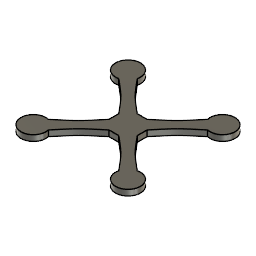
Drone 2 Polegadas (Autodesk Fusion 360 design; units mm, degrees)
Autodesk Fusion 360 part; units mm, degrees
note: some values were not read from the file. Set by a fixed rule: which sketch regions a step uses.
sketch "Esboço2" plane through (0, 0, 0) normal (0, 0, 1) x (1, 0, 0)
  circle A0 centre (-40.4, 40.4) radius 10.65
  circle A1 centre (40.4, 40.4) radius 10.65
  circle A2 centre (-40.4, -40.4) radius 10.65
  circle A3 centre (40.4, -40.4) radius 10.65
  line L0 (-40.4, 40.4) -> (-12.0945, 12.0945) construction
  line L1 (40.4, 40.4) -> (12.0945, 12.0945) construction
  line L2 (-40.4, -40.4) -> (-12.0945, -12.0945) construction
  line L3 (40.4, -40.4) -> (12.0945, -12.0945) construction
  line L4 (-6.0945, 12.0945) -> (6.0945, 12.0945)
  line L5 (12.0945, 6.0945) -> (12.0945, -6.0945)
  line L6 (6.0945, -12.0945) -> (-6.0945, -12.0945)
  line L7 (-12.0945, -6.0945) -> (-12.0945, 6.0945)
  line L8 (-30.0303, 37.9728) -> (-37.9728, 30.0303)
  line L9 (-37.9728, 30.0303) -> (-12.0945, 4.152) construction
  line L10 (-12.0945, 4.152) -> (-4.152, 12.0945) construction
  line L11 (-4.152, 12.0945) -> (-30.0303, 37.9728) construction
  line L12 (-17.0911, 25.0336) -> (-21.0624, 21.0624) construction
  spline S0 degree 2 poles (-30.0303, 37.9728) (-18.2817, 23.8431) (-4.152, 12.0945) knots 0 0 0 3.668443 3.668443 3.668443 weights 1 3 1
  spline S1 degree 2 poles (-37.9728, 30.0303) (-23.8431, 18.2817) (-12.0945, 4.152) knots 0 0 0 3.668443 3.668443 3.668443 weights 1 3 1
  line L13 (0, 12.0945) -> (0, -12.0945) construction
  spline S2 degree 2 poles (30.0303, 37.9728) (18.2817, 23.8431) (4.152, 12.0945) knots 0 0 0 3.668443 3.668443 3.668443 weights 1 3 1
  spline S3 degree 2 poles (37.9728, 30.0303) (23.8431, 18.2817) (12.0945, 4.152) knots 0 0 0 3.668443 3.668443 3.668443 weights 1 3 1
  line L14 (-12.0945, 0) -> (12.0945, 0) construction
  spline S4 degree 2 poles (-30.0303, -37.9728) (-18.2817, -23.8431) (-4.152, -12.0945) knots 0 0 0 3.668443 3.668443 3.668443 weights 1 3 1
  spline S5 degree 2 poles (-37.9728, -30.0303) (-23.8431, -18.2817) (-12.0945, -4.152) knots 0 0 0 3.668443 3.668443 3.668443 weights 1 3 1
  spline S6 degree 2 poles (30.0303, -37.9728) (18.2817, -23.8431) (4.152, -12.0945) knots 0 0 0 3.668443 3.668443 3.668443 weights 1 3 1
  spline S7 degree 2 poles (37.9728, -30.0303) (23.8431, -18.2817) (12.0945, -4.152) knots 0 0 0 3.668443 3.668443 3.668443 weights 1 3 1
  arc A4 (-6.0945, 12.0945) -> (-12.0945, 6.0945) centre (-6.0945, 6.0945) ccw
  arc A5 (12.0945, 6.0945) -> (6.0945, 12.0945) centre (6.0945, 6.0945) ccw
  arc A6 (-12.0945, -6.0945) -> (-6.0945, -12.0945) centre (-6.0945, -6.0945) ccw
  arc A7 (6.0945, -12.0945) -> (12.0945, -6.0945) centre (6.0945, -6.0945) ccw
  dimension "d49" = 80.8
  dimension "d50" = 80.8
  dimension "d51" = 21.3
  dimension "d52" = 21.3
  dimension "d53" = 21.3
  dimension "d54" = 21.3
  dimension "d55" = 114.2685
  dimension "d56" = 40.03
  dimension "d57" = 40.03
  dimension "d58" = 40.03
  dimension "d59" = 40.03
  dimension "d69" = 6
  dimension "d70" = 6
  dimension "d71" = 6
  dimension "d72" = 6
  constraint coincident A0.centre L0.start
  constraint coincident A1.centre L1.start
  constraint coincident A2.centre L2.start
  constraint coincident A3.centre L3.start
  constraint coincident A0 L8.start
  constraint coincident A0 L8.end
  constraint coincident L7 L9.end
  constraint coincident L4 L10.end
  constraint perpendicular L9 L10
  constraint coincident L0 L12.end
  constraint symmetric L0 L8.start L8.end
  constraint symmetric L0 L10.end L9.end
  constraint symmetric L0 S0 S1
  constraint perpendicular L6 L13
  constraint symmetric L8.start L13 S2.start
  constraint symmetric L10.end L13 S2.end
  constraint symmetric S0 L13 S2
  constraint symmetric L8.end L13 S3.start
  constraint symmetric L9.end L13 S3.end
  constraint symmetric S1 L13 S3
  constraint perpendicular L5 L14
  constraint symmetric L8.start L14 S4.start
  constraint symmetric L10.end L14 S4.end
  constraint symmetric S0 L14 S4
  constraint symmetric L8.end L14 S5.start
  constraint symmetric L9.end L14 S5.end
  constraint symmetric S1 L14 S5
  constraint symmetric S2.start L14 S6.start
  constraint symmetric S2.end L14 S6.end
  constraint symmetric S2 L14 S6
  constraint symmetric S3.start L14 S7.start
  constraint symmetric S3.end L14 S7.end
  constraint symmetric S3 L14 S7
  constraint coincident L4 L13.start
  constraint coincident L7 L14.start
  constraint coincident L0.end L4
  constraint coincident L0.end L7
  constraint tangent L4 A4
  constraint tangent L7 A4
  constraint coincident L5 L14.end
  constraint tangent L4 A5
  constraint tangent L5 A5
  constraint coincident L6 L13.end
  constraint tangent L6 A6
  constraint tangent L7 A6
  constraint coincident L3.end L5
  constraint coincident L3.end L6
  constraint tangent L5 A7
  constraint tangent L6 A7
  measures "d49" distance of A0.centre A1.centre
  measures "d50" distance of A0.centre A2.centre
  measures "d51" diameter of A0
  measures "d52" diameter of A1
  measures "d53" diameter of A2
  measures "d54" diameter of A3
  measures "d55" distance of A0.centre A3.centre
  measures "d56" distance of A0.centre L0.end
  measures "d57" distance of A1.centre L1.end
  measures "d58" distance of A2.centre L2.end
  measures "d59" distance of A3.centre L3.end
  measures "d69" radius of A4
  measures "d70" radius of A5
  measures "d71" radius of A6
  measures "d72" radius of A7
extrude "Extrusão1" add sketch "Esboço2" along normal blind 5
equation "d61 = 0.75"
equation "d62 = d61"
equation "d63 = d61"
equation "d64 = d62"
equation "d65 = d61"
equation "d66 = d62"
equation "d67 = d63"
equation "d68 = d64"
